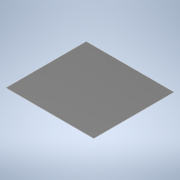
# Autodesk Inventor part: Sensor Placement Film
Saved by Autodesk Inventor 2022 (Build 260153000, 153)
## iProperties
Created: 2022-02-23
Part Number: Sensor Placement Film
Material: Thermoplastic Resin
Document SubType Name: Modeling
Designer: Caleb
Density: 1.28 g/cm^3
Appearance: Smooth - Black
Author: Caleb
Autodesk Inventor part; units mm, degrees
ref_plane "YZ Plane" through (0, 0, 0) normal (1, 0, 0) x (0, 1, 0)
ref_plane "XZ Plane" through (0, 0, 0) normal (0, 1, 0) x (-1, 0, 0)
ref_plane "XY Plane" through (0, 0, 0) normal (0, 0, 1) x (1, 0, 0)
sketch "Sketch1" plane through (0, 0, 0) normal (0, 1, 0) x (-1, 0, 0)
  line L0 (-23.3, -21.3) -> (23.3, -21.3)
  line L1 (23.3, -21.3) -> (23.3, 21.3)
  line L2 (23.3, 21.3) -> (-23.3, 21.3)
  line L3 (-23.3, 21.3) -> (-23.3, -21.3)
  line L4 (-23.3, -21.3) -> (23.3, 21.3) construction
  line L5 (23.3, -21.3) -> (-23.3, 21.3) construction
  point P0 (0, 0)
  dimension "d0" = 42.6
  dimension "d1" = 46.6
  constraints: 12 end point, 2 midpoint, 2 parallel, 1 horizontal, 1 perpendicular
  measures "d0" distance of L0.end L1.end
  measures "d1" distance of L1.end L2.end
extrude "Extrusion1" add sketch "Sketch1" along normal blind 0.08
body "Solid1"
